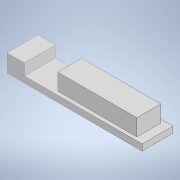
# Autodesk Inventor part: GPS
Saved by Autodesk Inventor 2020 (Build 240168000, 168)
## iProperties
Created: 2019-07-11
Part Number: GPS
Material: Generic
Document SubType Name: Modeling
Designer: tyrre
Density: 1 g/cm^3
Appearance: Default
Author: tyrre
Autodesk Inventor part; units mm, degrees
ref_plane "YZ Plane" through (0, 0, 0) normal (1, 0, 0) x (0, 1, 0)
ref_plane "XZ Plane" through (0, 0, 0) normal (0, 1, 0) x (-1, 0, 0)
ref_plane "XY Plane" through (0, 0, 0) normal (0, 0, 1) x (1, 0, 0)
sketch "Sketch4" plane through (0, 0, 0) normal (0, 0, 1) x (1, 0, 0)
  line L0 (-17.5, 0.8) -> (17.5, 0.8)
  line L1 (17.5, 0.8) -> (17.5, -0.8)
  line L2 (17.5, -0.8) -> (-17.5, -0.8)
  line L3 (-17.5, -0.8) -> (-17.5, 0.8)
  line L4 (-17.5, 0.8) -> (17.5, -0.8) construction
  line L5 (17.5, 0.8) -> (-17.5, -0.8) construction
  point P0 (0, 0)
  dimension "d4" = 35
  dimension "d5" = 1.6
  constraints: 12 end point, 2 midpoint, 2 parallel, 1 horizontal, 1 perpendicular
  measures "d4" distance of L1.end L2.end
  measures "d5" distance of L0.end L1.end
extrude "Extrusion2" add sketch "Sketch4" along normal mid plane 8
sketch "Sketch5" plane through (-17.5, 0.8, 4) normal (0, 1, 0) x (1, 0, 0)
  line L0 (35, 8) -> (35, 0) projected
  line L1 (35, 4) -> (32.75, 4)
  line L2 (32.75, 4) -> (12.25, 4)
  line L3 (12.25, 0.9) -> (32.75, 0.9)
  line L4 (32.75, 0.9) -> (32.75, 7.1)
  line L5 (32.75, 7.1) -> (12.25, 7.1)
  line L6 (12.25, 7.1) -> (12.25, 0.9)
  line L7 (12.25, 0.9) -> (32.75, 7.1) construction
  line L8 (32.75, 0.9) -> (12.25, 7.1) construction
  point P0 (17.5, 4)
  point P1 (22.5, 4)
  dimension "d8" = 2.25
  dimension "d9" = 20.5
  dimension "d10" = 20.5
  dimension "d11" = 6.2
  constraints: 16 end point, 4 midpoint, 3 horizontal, 2 parallel, 1 coincident, 1 perpendicular
  measures "d8" distance of L1.start L1.end
  measures "d9" distance of L2.start L2.end
  measures "d10" distance of L5.end L4.end
  measures "d11" distance of L4.end L3.end
extrude "Extrusion3" add sketch "Sketch5" along normal blind 4.3
sketch "Sketch6" plane through (-17.5, 0.8, 4) normal (0, 1, 0) x (1, 0, 0)
  line L0 (32.75, 0.9) -> (12.25, 0.9) projected
  line L1 (12.25, 0.9) -> (12.25, 7.1) projected
  line L2 (12.25, 7.1) -> (32.75, 7.1) projected
  line L3 (32.75, 7.1) -> (32.75, 0.9) projected
  line L4 (0, 8) -> (0, 0) projected
  line L5 (35, 0) -> (0, 0) projected
  line L6 (35, 0) -> (35, 8) projected
  line L7 (0, 8) -> (35, 8) projected
  line L8 (0, 8) -> (0, 0) projected
  line L9 (0, 0) -> (0, 8)
  line L10 (0, 8) -> (4.5, 8)
  line L11 (4.5, 8) -> (4.5, 0)
  line L12 (4.5, 0) -> (0, 0)
  point P0 (17.5, 4)
  dimension "d14" = 4.5
  constraints: 8 end point, 3 equal length, 1 perpendicular
  measures "d14" distance of L4.start L10.end
extrude "Extrusion4" add sketch "Sketch6" along normal blind 2.95 separate body contours L7 L11 L5 L4
body "Solid2"
body "Solid3"
